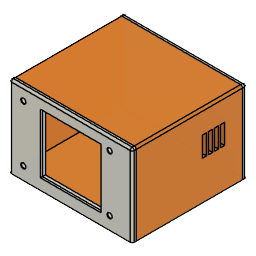
AirLog-E(together, no-placeholder-components) (Autodesk Fusion 360 design; units mm, degrees)
Autodesk Fusion 360 part; units mm, degrees
note: some values were not read from the file. Chosen so that the rebuilt part matches the saved one: which sketch regions a step uses; that a step has no effect.
sketch "Sketch1" plane through (0, 0, 0) normal (0, 1, 0) x (1, 0, 0)
  line L0 (24.9, -1.7) -> (-4.3, -1.7)
  line L1 (-4.3, -1.7) -> (-4.3, -30.3)
  line L2 (-4.3, -30.3) -> (24.9, -30.3)
  line L3 (24.9, -30.3) -> (24.9, -1.7)
  line L4 (30.9, 4.3) -> (-10.3, 4.3)
  line L5 (-10.3, -36.3) -> (30.9, -36.3)
  line L6 (-10.3, -36.3) -> (-20.3, -36.3)
  line L7 (-10.3, 4.3) -> (-20.3, 4.3)
  line L8 (30.9, -36.3) -> (40.9, -36.3)
  line L9 (30.9, 4.3) -> (40.9, 4.3)
  line L10 (40.9, -36.3) -> (40.9, 4.3)
  line L11 (-20.3, -36.3) -> (-20.3, 4.3)
  circle A0 centre (-13.355, -30.08) radius 1.08
  circle A1 centre (29.645, -30.08) radius 1.08
  circle A2 centre (-13.355, -2.08) radius 1.08
  circle A3 centre (29.645, -2.08) radius 1.08
  dimension "d2" = 6
  dimension "d3" = 10
  dimension "d4" = 10
  dimension "d5" = 10
  dimension "d6" = 10
  measures "d3" distance of L5.start L6.end
  measures "d4" distance of L4.end L7.end
  measures "d5" distance of L5.end L8.end
  measures "d6" distance of L4.start L9.end
extrude "Extrude1" add sketch "Sketch1" along normal blind 2 makes body 1
sketch "Sketch2" plane through (0, 0, 0) normal (0, 1, 0) x (1, 0, 0)
  circle A0 centre (29.635, -30.08) radius 1.0801
  circle A1 centre (-13.36, -30.08) radius 1.08
  circle A2 centre (-13.355, -2.08) radius 1.08
  circle A3 centre (29.6413, -2.0788) radius 1.0788
  line L0 (29.65, -29) -> (29.65, -28) construction
  line L1 (28.56, -30.08) -> (27.56, -30.08) construction
  line L2 (30.7151, -30.08) -> (31.7151, -30.08) construction
  line L3 (31.7151, -30.08) -> (31.7151, -28)
  line L4 (31.7151, -28) -> (29.65, -28)
  line L5 (27.56, -30.08) -> (27.56, -28)
  line L6 (27.56, -28) -> (29.65, -28)
  line L7 (27.56, -30.08) -> (27.56, -36.3)
  line L8 (31.7151, -30.08) -> (31.7151, -36.3)
  line L9 (31.7151, -36.3) -> (27.56, -36.3)
  line L10 (-15.44, -30.08) -> (-15.44, -36.3)
  line L11 (-15.44, -28) -> (-13.35, -28)
  line L12 (-11.2849, -36.3) -> (-15.44, -36.3)
  line L13 (-11.2849, -28) -> (-13.35, -28)
  line L14 (-14.44, -30.08) -> (-15.44, -30.08) construction
  line L15 (-11.2849, -30.08) -> (-11.2849, -36.3)
  line L16 (-13.35, -29) -> (-13.35, -28) construction
  circle A4 centre (-13.365, -30.08) radius 1.0801
  line L17 (-12.2849, -30.08) -> (-11.2849, -30.08) construction
  line L18 (-11.2849, -30.08) -> (-11.2849, -28)
  line L19 (-15.44, -30.08) -> (-15.44, -28)
  line L20 (-13.35, -3.15) -> (-13.35, -4.15) construction
  line L21 (-15.4151, -2.07) -> (-15.4151, 4.15)
  line L22 (-11.26, -2.07) -> (-11.26, 4.15)
  line L23 (-15.4151, -2.07) -> (-15.4151, -4.15)
  line L24 (-15.4151, -4.15) -> (-13.35, -4.15)
  line L25 (-11.26, -2.07) -> (-11.26, -4.15)
  line L26 (-14.4151, -2.07) -> (-15.4151, -2.07) construction
  line L27 (-11.26, -4.15) -> (-13.35, -4.15)
  circle A5 centre (-13.335, -2.07) radius 1.0801
  line L28 (-12.26, -2.07) -> (-11.26, -2.07) construction
  circle A6 centre (-13.34, -2.07) radius 1.08
  line L29 (28.5849, -2.07) -> (27.5849, -2.07) construction
  line L30 (31.74, -4.15) -> (29.65, -4.15)
  circle A7 centre (29.645, -2.08) radius 1.08
  line L31 (31.74, -2.07) -> (31.74, -4.15)
  line L32 (31.74, -2.07) -> (31.74, 4.15)
  line L33 (27.5849, -2.07) -> (27.5849, -4.15)
  line L34 (27.5849, -4.15) -> (29.65, -4.15)
  line L35 (30.74, -2.07) -> (31.74, -2.07) construction
  line L36 (27.5849, -2.07) -> (27.5849, 4.15)
  line L37 (29.65, -3.15) -> (29.65, -4.15) construction
  circle A8 centre (29.665, -2.07) radius 1.0801
  circle A9 centre (29.66, -2.07) radius 1.08
  line L38 (31.7151, -36.3) -> (40.9, -36.3)
  line L39 (40.9, -36.3) -> (40.9, 4.3)
  line L40 (40.9, 4.3) -> (-20.3, 4.3)
  line L41 (-20.3, 4.3) -> (-20.3, -36.3)
  line L42 (-20.3, -36.3) -> (27.56, -36.3)
  line L43 (31.74, 4.15) -> (31.74, 4.3)
  line L44 (27.5849, 4.15) -> (27.5849, 4.3)
  line L45 (-11.26, 4.15) -> (-11.26, 4.3)
  line L46 (-15.4151, 4.15) -> (-15.4151, 4.3)
  line L47 (31.7151, -33.8) -> (27.56, -33.8)
  line L48 (-17.8, -33.8) -> (27.56, -33.8)
  line L49 (-17.8, 1.8) -> (-17.8, -33.8)
  line L50 (38.4, 1.8) -> (-17.8, 1.8)
  line L51 (38.4, -33.8) -> (38.4, 1.8)
  line L52 (31.7151, -33.8) -> (38.4, -33.8)
  dimension "d9" = 1
  dimension "d10" = 1
  dimension "d11" = 1
  dimension "d12" = 1
  dimension "d13" = 1
  dimension "d14" = 1
  dimension "d15" = 1
  dimension "d16" = 1
  dimension "d17" = 2.5
  constraint coincident A0 L0.start
  constraint vertical L0
  constraint horizontal L1
  constraint coincident A0 L2.start
  constraint parallel L1 L2
  constraint perpendicular L2 L3
  constraint perpendicular L1 L5
  constraint perpendicular L0 L6
  constraint perpendicular L1 L7
  constraint perpendicular L2 L8
  constraint perpendicular L7 L9
  constraint coincident L16.start A4
  constraint vertical L16
  constraint horizontal L14
  constraint coincident L17.start A4
  constraint parallel L14 L17
  constraint perpendicular L17 L18
  constraint perpendicular L14 L19
  constraint perpendicular L11 L16
  constraint perpendicular L10 L14
  constraint perpendicular L15 L17
  constraint perpendicular L10 L12
  constraint coincident L20.start A5
  constraint coincident L26.start A5
  constraint parallel L26 L28
  constraint perpendicular L23 L26
  constraint perpendicular L25 L28
  constraint perpendicular L20 L27
  constraint perpendicular L22 L28
  constraint perpendicular L21 L26
  constraint coincident L37.start A8
  constraint coincident L29.start A8
  constraint parallel L29 L35
  constraint perpendicular L29 L33
  constraint perpendicular L31 L35
  constraint perpendicular L30 L37
  constraint perpendicular L32 L35
  constraint perpendicular L29 L36
  constraint perpendicular L8 L38
  constraint perpendicular L38 L39
  constraint perpendicular L21 L40
  constraint perpendicular L40 L41
  constraint perpendicular L7 L42
  constraint coincident L40 L43.end
  constraint perpendicular L40 L43
  constraint coincident L40 L44.end
  constraint perpendicular L40 L44
  constraint coincident L40 L45.end
  constraint perpendicular L40 L45
  constraint coincident L40 L46.end
  constraint perpendicular L40 L46
  measures "d9" distance of L1.start L1.end
  measures "d10" distance of L2.start L2.end
  measures "d11" distance of L10.start L14.start
  measures "d12" distance of L15.start L17.start
  measures "d13" distance of L22.start L28.start
  measures "d14" distance of L21.start L26.start
  measures "d15" distance of L31.start L35.start
  measures "d16" distance of L29.end L29.start
extrude "Extrude2" add sketch "Sketch2" along normal blind 50 separate body contours L3 L4 L5 L6 L7 L8 L47 | L8 L32 L38 L39 L40 L43 L50 L51 L52 | L7 L8 L9 L47 | L7 L15 L42 L48 | L10 L11 L13 L15 L18 L19 L48 | L10 L12 L15 L42 L48 | L10 L21 L40 L41 L42 L46 L48 L49 L50 | L32 L36 L40 L43 L44 L50 | L30 L31 L32 L33 L34 L36 L50 | L22 L36 L40 L44 L45 L50 | L21 L22 L40 L45 L46 L50 | L21 L22 L23 L24 L25 L27 L50 makes body 2
move_body "Move1" bodies 2 to x (1, 0, 0) y (0, 1, 0) z (0, 0, 1) at (0, 5, 0)
sketch "Sketch3" plane through (0, 5, 0) normal (0, -1, 0) x (1, 0, 0)
  line L0 (31.7151, 28) -> (31.7151, 33.8)
  line L1 (31.7151, 33.8) -> (38.4, 33.8)
  line L2 (38.4, 33.8) -> (38.4, -1.8)
  line L3 (38.4, -1.8) -> (31.74, -1.8)
  line L4 (31.74, -1.8) -> (31.74, 4.15)
  line L5 (31.74, 4.15) -> (29.65, 4.15)
  line L6 (29.65, 4.15) -> (27.5849, 4.15)
  line L7 (27.5849, 4.15) -> (27.5849, -1.8)
  line L8 (27.5849, -1.8) -> (-11.26, -1.8)
  line L9 (-11.26, -1.8) -> (-11.26, 4.15)
  line L10 (-11.26, 4.15) -> (-13.35, 4.15)
  line L11 (-13.35, 4.15) -> (-15.4151, 4.15)
  line L12 (-15.4151, 4.15) -> (-15.4151, -1.8)
  line L13 (-15.4151, -1.8) -> (-17.8, -1.8)
  line L14 (-17.8, -1.8) -> (-17.8, 33.8)
  line L15 (-17.8, 33.8) -> (-15.44, 33.8)
  line L16 (-15.44, 33.8) -> (-15.44, 28)
  line L17 (-15.44, 28) -> (-13.35, 28)
  line L18 (-13.35, 28) -> (-11.2849, 28)
  line L19 (-11.2849, 28) -> (-11.2849, 33.8)
  line L20 (-11.2849, 33.8) -> (27.56, 33.8)
  line L21 (27.56, 33.8) -> (27.56, 28)
  line L22 (27.56, 28) -> (29.65, 28)
  line L23 (29.65, 28) -> (31.7151, 28)
  circle A0 centre (29.635, 30.08) radius 1.0801
  arc A1 (-13.9461, 1.1761) -> (-13.36, 0.9902) centre (-13.34, 2.07) ccw
  arc A2 (-12.8659, 3.0429) -> (-13.9461, 1.1761) centre (-13.355, 2.08) ccw
  arc A3 (-13.36, 0.9902) -> (-12.8659, 3.0429) centre (-13.335, 2.07) ccw
  arc A4 (29.64, 0.9902) -> (30.1341, 3.0429) centre (29.665, 2.07) ccw
  arc A5 (29.1359, 1.1257) -> (29.64, 0.9902) centre (29.66, 2.07) ccw
  arc A6 (28.9927, 2.9408) -> (29.1359, 1.1257) centre (29.6413, 2.0788) ccw
  arc A7 (30.1341, 3.0429) -> (28.9927, 2.9408) centre (29.645, 2.08) ccw
  arc A8 (-13.34, 29.0002) -> (-13.34, 31.1598) centre (-13.36, 30.08) ccw
  arc A9 (-13.34, 31.1598) -> (-13.34, 29.0002) centre (-13.365, 30.08) ccw
  line L24 (40.9, 36.3) -> (-20.3, 36.3)
  line L25 (-20.3, 36.3) -> (-20.3, -4.3)
  line L26 (-20.3, -4.3) -> (40.9, -4.3)
  line L27 (40.9, -4.3) -> (40.9, 36.3)
  line L28 (-20.3, 36.3) -> (40.9, 36.3)
  line L29 (40.9, 36.3) -> (40.9, -4.3)
  line L30 (40.9, -4.3) -> (-20.3, -4.3)
  line L31 (-20.3, -4.3) -> (-20.3, 36.3)
  line L32 (38.4, -1.8) -> (-17.8, -1.8)
  line L33 (-17.8, -1.8) -> (-17.8, 33.8)
  line L34 (-17.8, 33.8) -> (38.4, 33.8)
  line L35 (38.4, 33.8) -> (38.4, -1.8)
  constraint horizontal L28
  constraint vertical L29
  constraint horizontal L30
  constraint vertical L31
  constraint coincident L26.end L27.start
  constraint coincident L24.end L25.start
  constraint horizontal L32
  constraint vertical L33
  constraint horizontal L34
  constraint vertical L35
  constraint coincident L14.end L15.start
  constraint coincident L2.end L3.start
extrude "Extrude3" add sketch "Sketch3" along normal blind 3 contours L24 L25 L26 L27 L28 L29 L30 L31 bodies 2
sketch "Sketch4" plane through (0, 55, 0) normal (0, 1, 0) x (-1, 0, 0)
  line L0 (-31.7151, 33.8) -> (-31.7151, 28)
  line L1 (-31.7151, 28) -> (-29.65, 28)
  line L2 (-29.65, 28) -> (-27.56, 28)
  line L3 (-27.56, 28) -> (-27.56, 33.8)
  line L4 (-27.56, 33.8) -> (11.2849, 33.8)
  line L5 (11.2849, 33.8) -> (11.2849, 28)
  line L6 (11.2849, 28) -> (13.35, 28)
  line L7 (13.35, 28) -> (15.44, 28)
  line L8 (15.44, 28) -> (15.44, 33.8)
  line L9 (15.44, 33.8) -> (17.8, 33.8)
  line L10 (17.8, 33.8) -> (17.8, -1.8)
  line L11 (17.8, -1.8) -> (15.4151, -1.8)
  line L12 (15.4151, -1.8) -> (15.4151, 4.15)
  line L13 (15.4151, 4.15) -> (13.35, 4.15)
  line L14 (13.35, 4.15) -> (11.26, 4.15)
  line L15 (11.26, 4.15) -> (11.26, -1.8)
  line L16 (11.26, -1.8) -> (-27.5849, -1.8)
  line L17 (-27.5849, -1.8) -> (-27.5849, 4.15)
  line L18 (-27.5849, 4.15) -> (-29.65, 4.15)
  line L19 (-29.65, 4.15) -> (-31.74, 4.15)
  line L20 (-31.74, 4.15) -> (-31.74, -1.8)
  line L21 (-31.74, -1.8) -> (-38.4, -1.8)
  line L22 (-38.4, -1.8) -> (-38.4, 33.8)
  line L23 (-38.4, 33.8) -> (-31.7151, 33.8)
  circle A0 centre (-29.635, 30.08) radius 1.0801
  arc A1 (13.36, 0.9902) -> (13.9461, 1.1761) centre (13.34, 2.07) ccw
  arc A2 (12.8659, 3.0429) -> (13.36, 0.9902) centre (13.335, 2.07) ccw
  arc A3 (13.9461, 1.1761) -> (12.8659, 3.0429) centre (13.355, 2.08) ccw
  arc A4 (-30.1341, 3.0429) -> (-29.64, 0.9902) centre (-29.665, 2.07) ccw
  arc A5 (-28.9927, 2.9408) -> (-30.1341, 3.0429) centre (-29.645, 2.08) ccw
  arc A6 (-29.1359, 1.1257) -> (-28.9927, 2.9408) centre (-29.6413, 2.0788) ccw
  arc A7 (-29.64, 0.9902) -> (-29.1359, 1.1257) centre (-29.66, 2.07) ccw
  arc A8 (13.34, 31.1598) -> (13.34, 29.0002) centre (13.36, 30.08) ccw
  arc A9 (13.34, 29.0002) -> (13.34, 31.1598) centre (13.365, 30.08) ccw
  line L24 (20.3, 36.3) -> (-40.9, 36.3)
  line L25 (-40.9, 36.3) -> (-40.9, -4.3)
  line L26 (-40.9, -4.3) -> (20.3, -4.3)
  line L27 (20.3, -4.3) -> (20.3, 36.3)
  line L28 (-31.7151, 33.8) -> (-27.56, 33.8)
  line L29 (-27.56, 33.8) -> (-27.56, 28)
  line L30 (-27.56, 28) -> (-31.7151, 28)
  line L31 (-31.7151, 28) -> (-31.7151, 33.8)
  line L32 (11.2849, 33.8) -> (15.44, 33.8)
  line L33 (15.44, 33.8) -> (15.44, 28)
  line L34 (15.44, 28) -> (11.2849, 28)
  line L35 (11.2849, 28) -> (11.2849, 33.8)
  line L36 (11.26, 4.15) -> (15.4151, 4.15)
  line L37 (15.4151, 4.15) -> (15.4151, -1.8)
  line L38 (15.4151, -1.8) -> (11.26, -1.8)
  line L39 (11.26, -1.8) -> (11.26, 4.15)
  line L40 (-31.74, 4.15) -> (-27.5849, 4.15)
  line L41 (-27.5849, 4.15) -> (-27.5849, -1.8)
  line L42 (-27.5849, -1.8) -> (-31.74, -1.8)
  line L43 (-31.74, -1.8) -> (-31.74, 4.15)
  constraint horizontal L28
  constraint vertical L29
  constraint horizontal L30
  constraint vertical L31
  constraint coincident L2.end L3.start
  constraint coincident L0.start L23.end
  constraint horizontal L32
  constraint vertical L33
  constraint horizontal L34
  constraint vertical L35
  constraint coincident L7.end L8.start
  constraint coincident L4.end L5.start
  constraint horizontal L36
  constraint vertical L37
  constraint horizontal L38
  constraint vertical L39
  constraint coincident L11.end L12.start
  constraint coincident L14.end L15.start
  constraint horizontal L40
  constraint vertical L41
  constraint horizontal L42
  constraint vertical L43
  constraint coincident L16.end L17.start
  constraint coincident L19.end L20.start
extrude "Extrude4" cut sketch "Sketch4" against normal blind 48 contours L0 L1 L2 L3 L28 L29 L30 L31 | L5 L6 L7 L8 L32 L33 L34 L35 | L17 L18 L19 L20 L40 L41 L42 L43 | L12 L13 L14 L15 L36 L37 L38 L39 | A0 | A1 A2 A3 | A4 A5 A6 A7 | A8 A9 bodies 2
chamfer "Chamfer1" distance 0.2 angle 45 10 edges at (-12.28, 5, 30.08) (-14.4451, 5, 30.08) (28.628, 5, 29.6894) (30.7151, 5, 1.8172) (28.5658, 5, 1.9939) (29.3796, 5, 1.027) (29.5487, 5, 3.1557) (-12.2849, 5, 1.8172) (-13.6665, 5, 1.0405) (-14.2898, 5, 2.6209) on bodies 2
chamfer "Chamfer2" distance 0.2 angle 45 4 edges at (-14.3619, 0, 29.6895) (28.6381, 0, 1.6895) (28.6381, 0, 29.6895) (-14.3619, 0, 1.6895) on bodies 1
chamfer "Chamfer3" distance 0.5 angle 45 4 edges at (-4.3, 0, 16) (10.3, 0, 30.3) (10.3, 0, 1.7) (24.9, 0, 16) on bodies 1
sketch "Sketch5" plane through (0, 0, 0) normal (0, 0, 1) x (1, 0, 0)
  line L0 (20, -25) -> (-30, -25)
  line L1 (-30, -25) -> (-30, 9)
  line L2 (-30, 9) -> (20, 9)
  line L3 (20, 9) -> (20, -25)
  dimension "d27" = 34
  constraint horizontal L0
  constraint vertical L1
  constraint horizontal L2
  constraint vertical L3
  measures "d27" distance of L0.start L2.end
sketch "Sketch6" plane through (0, 0, 10) normal (0, 0, 1) x (-1, 0, 0)
  line L0 (-17, 21) -> (-17, -5)
  line L1 (-17, -5) -> (27, -5)
  line L2 (27, -5) -> (27, 21)
  line L3 (27, 21) -> (-17, 21)
  line L4 (12.4645, 11) -> (-7, 11) construction
  line L5 (-7, 11) -> (-7, 4.44) construction
  line L6 (-7, 4.44) -> (12.4645, 4.44) construction
  line L7 (12.4645, 4.44) -> (12.4645, 11) construction
  dimension "d38" = 2
sketch "Sketch7" plane through (-17.8, 0, 0) normal (1, 0, 0) x (0, 1, 0)
  line L0 (2, -1.8) -> (55, -1.8)
  line L1 (55, -1.8) -> (55, 33.8)
  line L2 (55, 33.8) -> (2, 33.8)
  line L3 (2, 33.8) -> (2, -1.8)
  line L4 (30, 25) -> (32, 25)
  line L5 (32, 25) -> (32, 20)
  line L6 (32, 20) -> (30, 20)
  line L7 (30, 20) -> (30, 25)
  constraint horizontal L4
  constraint vertical L5
  constraint horizontal L6
  constraint vertical L7
extrude "Extrude7" add sketch "Sketch7" along normal blind 8 contours L4 L5 L6 L7 bodies 2
sketch "Sketch8" plane through (0, 32, 0) normal (0, 1, 0) x (-1, 0, 0)
  line L0 (17.8, 20) -> (17.8, 25)
  line L1 (17.8, 25) -> (9.8, 25)
  line L2 (9.8, 25) -> (9.8, 20)
  line L3 (9.8, 20) -> (17.8, 20)
  circle A0 centre (13.5, 22.5) radius 1.25
  dimension "d44" = 2.5
  measures "d44" diameter of A0
extrude "Extrude8" cut sketch "Sketch8" against normal blind 2 contours A0 bodies 2
sketch "Sketch9" plane through (38.4, 0, 0) normal (-1, 0, 0) x (0, -1, 0)
  line L0 (-2, 33.8) -> (-55, 33.8)
  line L1 (-55, 33.8) -> (-55, -1.8)
  line L2 (-55, -1.8) -> (-2, -1.8)
  line L3 (-2, -1.8) -> (-2, 33.8)
  line L4 (-30, 25) -> (-30, 20)
  line L5 (-30, 20) -> (-32, 20)
  line L6 (-32, 25) -> (-30, 25)
  line L7 (-32, 20) -> (-32, 25)
  constraint horizontal L6
  constraint vertical L4
  constraint horizontal L5
  constraint vertical L7
extrude "Extrude9" add sketch "Sketch9" along normal blind 8 contours L4 L5 L6 L7 bodies 2
sketch "Sketch10" plane through (0, 32, 0) normal (0, 1, 0) x (-1, 0, 0)
  line L0 (-38.4, 25) -> (-38.4, 20)
  line L1 (-38.4, 20) -> (-30.4, 20)
  line L2 (-30.4, 20) -> (-30.4, 25)
  line L3 (-30.4, 25) -> (-38.4, 25)
  circle A0 centre (-34.1, 22.5) radius 1.25
  dimension "d51" = 2.5
  measures "d51" diameter of A0
extrude "Extrude10" cut sketch "Sketch10" against normal blind 2 contours A0 bodies 2
sketch "Sketch11" plane through (-20.3, 0, 0) normal (-1, 0, 0) x (0, -1, 0)
  line L0 (-2, 36.3) -> (-55, 36.3)
  line L1 (-55, 36.3) -> (-55, -4.3)
  line L2 (-55, -4.3) -> (-2, -4.3)
  line L3 (-2, -4.3) -> (-2, 36.3)
  line L4 (-35, 25) -> (-37, 25)
  line L5 (-37, 25) -> (-37, 15)
  line L6 (-37, 15) -> (-35, 15)
  line L7 (-35, 15) -> (-35, 25)
  line L8 (-38, 25) -> (-40, 25)
  line L9 (-40, 25) -> (-40, 15)
  line L10 (-40, 15) -> (-38, 15)
  line L11 (-38, 15) -> (-38, 25)
  line L12 (-41, 25) -> (-43, 25)
  line L13 (-43, 25) -> (-43, 15)
  line L14 (-43, 15) -> (-41, 15)
  line L15 (-41, 15) -> (-41, 25)
  line L16 (-44, 25) -> (-46, 25)
  line L17 (-46, 25) -> (-46, 15)
  line L18 (-46, 15) -> (-44, 15)
  line L19 (-44, 15) -> (-44, 25)
  dimension "d54" = 2
  dimension "d55" = 10
  dimension "d56" = 2
  dimension "d57" = 10
  dimension "d58" = 2
  dimension "d59" = 10
  dimension "d60" = 2
  dimension "d61" = 10
  constraint horizontal L4
  constraint vertical L5
  constraint horizontal L6
  constraint vertical L7
  constraint horizontal L8
  constraint vertical L9
  constraint horizontal L10
  constraint vertical L11
  constraint horizontal L12
  constraint vertical L13
  constraint horizontal L14
  constraint vertical L15
  constraint horizontal L16
  constraint vertical L17
  constraint horizontal L18
  constraint vertical L19
  measures "d54" distance of L4.start L4.end
  measures "d55" distance of L4.start L6.end
  measures "d56" distance of L8.start L8.end
  measures "d57" distance of L8.start L10.end
  measures "d58" distance of L12.start L12.end
  measures "d59" distance of L12.start L14.end
  measures "d60" distance of L16.start L16.end
  measures "d61" distance of L16.start L18.end
sketch "Sketch12" plane through (40.9, 0, 0) normal (1, 0, 0) x (0, 1, 0)
  line L0 (2, -4.3) -> (55, -4.3)
  line L1 (55, -4.3) -> (55, 36.3)
  line L2 (55, 36.3) -> (2, 36.3)
  line L3 (2, 36.3) -> (2, -4.3)
  line L4 (41, 25) -> (41, 15)
  line L5 (46, 25) -> (44, 25)
  line L6 (40, 15) -> (40, 25)
  line L7 (43, 15) -> (43, 25)
  line L8 (41, 15) -> (43, 15)
  line L9 (43, 25) -> (41, 25)
  line L10 (37, 25) -> (35, 25)
  line L11 (38, 25) -> (38, 15)
  line L12 (37, 15) -> (37, 25)
  line L13 (46, 15) -> (46, 25)
  line L14 (38, 15) -> (40, 15)
  line L15 (35, 25) -> (35, 15)
  line L16 (44, 15) -> (46, 15)
  line L17 (44, 25) -> (44, 15)
  line L18 (35, 15) -> (37, 15)
  line L19 (40, 25) -> (38, 25)
  dimension "d62" = 2
  dimension "d63" = 10
  dimension "d64" = 2
  dimension "d65" = 10
  dimension "d66" = 2
  dimension "d67" = 10
  dimension "d68" = 2
  dimension "d69" = 10
  constraint horizontal L5
  constraint vertical L17
  constraint horizontal L16
  constraint vertical L13
  constraint horizontal L9
  constraint vertical L4
  constraint horizontal L8
  constraint vertical L7
  constraint horizontal L19
  constraint vertical L11
  constraint horizontal L14
  constraint vertical L6
  constraint horizontal L10
  constraint vertical L15
  constraint horizontal L18
  constraint vertical L12
  measures "d62" distance of L5.end L5.start
  measures "d63" distance of L5.start L13.start
  measures "d64" distance of L7.end L4.start
  measures "d65" distance of L7.end L7.start
  measures "d66" distance of L11.start L6.end
  measures "d67" distance of L6.start L6.end
  measures "d68" distance of L10.start L10.end
  measures "d69" distance of L10.start L12.start
extrude "Extrude11" cut sketch "Sketch11" against normal blind 2.5 contours L4 L5 L6 L7 | L8 L9 L10 L11 | L12 L13 L14 L15 | L16 L17 L18 L19 bodies 2
extrude "Extrude12" cut sketch "Sketch12" against normal blind 2.5 contours L4 L7 L8 L9 | L5 L13 L16 L17 | L6 L11 L14 L19 | L10 L12 L15 L18 bodies 2
sketch "Sketch13" plane through (0, 0, 0) normal (0, 1, 0) x (1, 0, 0)
  line L0 (40.9, -36.3, 55) -> (-20.3, -36.3, 55)
  line L1 (-20.3, -36.3, 55) -> (-20.3, 4.3, 55)
  line L2 (-20.3, 4.3, 55) -> (40.9, 4.3, 55)
  line L3 (40.9, 4.3, 55) -> (40.9, -36.3, 55)
  line L4 (31.7151, -36.3, 55) -> (27.56, -36.3, 55)
  line L5 (29.65, -29, 55) -> (29.65, -28, 55) construction
  line L6 (27.5849, 4.15, 55) -> (27.5849, 4.3, 55)
  line L7 (30.74, -2.07, 55) -> (31.74, -2.07, 55) construction
  line L8 (29.65, -3.15, 55) -> (29.65, -4.15, 55) construction
  line L9 (-17.8, -33.8, 55) -> (27.56, -33.8, 55)
  line L10 (-14.4151, -2.07, 55) -> (-15.4151, -2.07, 55) construction
  line L11 (-13.35, -29, 55) -> (-13.35, -28, 55) construction
  line L12 (-14.44, -30.08, 55) -> (-15.44, -30.08, 55) construction
  line L13 (28.56, -30.08, 55) -> (27.56, -30.08, 55) construction
  line L14 (-11.2849, -36.3, 55) -> (-15.44, -36.3, 55)
  line L15 (30.7151, -30.08, 55) -> (31.7151, -30.08, 55) construction
  line L16 (40.9, 4.3, 55) -> (-20.3, 4.3, 55)
  line L17 (38.4, 1.8, 55) -> (-17.8, 1.8, 55)
  line L18 (-20.3, 4.3, 55) -> (-20.3, -36.3, 55)
  line L19 (-12.26, -2.07, 55) -> (-11.26, -2.07, 55) construction
  line L20 (-15.4151, 4.15, 55) -> (-15.4151, 4.3, 55)
  line L21 (-11.26, 4.15, 55) -> (-11.26, 4.3, 55)
  line L22 (-12.2849, -30.08, 55) -> (-11.2849, -30.08, 55) construction
  line L23 (-13.35, -3.15, 55) -> (-13.35, -4.15, 55) construction
  line L24 (-20.3, -36.3, 55) -> (27.56, -36.3, 55)
  line L25 (-17.8, 1.8, 55) -> (-17.8, -33.8, 55)
  line L26 (38.4, -33.8, 55) -> (38.4, 1.8, 55)
  line L27 (31.7151, -33.8, 55) -> (38.4, -33.8, 55)
  line L28 (31.7151, -33.8, 55) -> (27.56, -33.8, 55)
  line L29 (31.74, 4.15, 55) -> (31.74, 4.3, 55)
  line L30 (28.5849, -2.07, 55) -> (27.5849, -2.07, 55) construction
  line L31 (40.9, -36.3, 55) -> (40.9, 4.3, 55)
  line L32 (31.7151, -36.3, 55) -> (40.9, -36.3, 55)
  circle A0 through (31.635, -30.08, 55) (28.635, -28.348, 55) (28.635, -31.8121, 55)
  circle A1 through (-11.365, -30.08, 55) (-14.365, -28.348, 55) (-14.365, -31.8121, 55)
  circle A2 through (-11.34, -2.07, 55) (-14.34, -0.3379, 55) (-14.34, -3.802, 55)
  circle A3 through (31.645, -2.08, 55) (28.645, -0.3479, 55) (28.645, -3.8121, 55)
  line L33 (31.74, -1.2617, 55) -> (33.24, -1.2617, 55) construction
  line L34 (27.5849, -1.1744, 55) -> (26.0849, -1.1744, 55) construction
  line L35 (29.65, -4.15, 55) -> (29.65, -5.65, 55) construction
  line L36 (33.24, -1.2617, 55) -> (33.24, 1.8, 55)
  line L37 (26.0849, -1.1744, 55) -> (26.0849, 1.8, 55)
  line L38 (29.65, -5.65, 55) -> (33.24, -5.65, 55)
  line L39 (29.65, -5.65, 55) -> (26.0849, -5.65, 55)
  line L40 (26.0849, -5.65, 55) -> (26.0849, -1.1744, 55)
  line L41 (33.24, -5.65, 55) -> (33.24, -1.2617, 55)
  line L42 (-13.35, -4.07, 55) -> (-13.35, -5.57, 55) construction
  line L43 (-15.34, -2.07, 55) -> (-16.84, -2.07, 55) construction
  line L44 (-11.26, -2.07, 55) -> (-9.76, -2.07, 55) construction
  line L45 (-13.35, -5.57, 55) -> (-9.76, -5.57, 55)
  line L46 (-13.35, -5.57, 55) -> (-16.84, -5.57, 55)
  line L47 (-16.84, -5.57, 55) -> (-16.84, 1.8, 55)
  line L48 (-9.76, -5.57, 55) -> (-9.76, 1.8, 55)
  line L49 (-11.365, -30.08, 55) -> (-9.865, -30.08, 55) construction
  line L50 (-15.365, -30.08, 55) -> (-16.865, -30.08, 55) construction
  line L51 (-13.35, -28.0801, 55) -> (-13.35, -26.5801, 55) construction
  line L52 (-16.865, -30.08, 55) -> (-16.865, -30, 55) construction
  line L53 (-9.865, -30.08, 55) -> (-9.865, -33.8, 55)
  line L54 (-16.865, -30.08, 55) -> (-16.865, -33.8, 55)
  line L55 (-13.35, -26.5801, 55) -> (-16.865, -26.5801, 55)
  line L56 (-13.35, -26.5801, 55) -> (-9.865, -26.5801, 55)
  line L57 (-9.865, -26.5801, 55) -> (-9.865, -29.5, 55)
  line L58 (-16.865, -26.5801, 55) -> (-16.865, -30.08, 55)
  line L59 (27.635, -30.08, 55) -> (26.135, -30.08, 55) construction
  line L60 (31.635, -30.08, 55) -> (33.135, -30.08, 55) construction
  line L61 (29.65, -28.0801, 55) -> (29.65, -26.5801, 55) construction
  line L62 (26.135, -30.08, 55) -> (26.135, -33.8, 55)
  line L63 (33.135, -30.08, 55) -> (33.135, -33.8, 55)
  line L64 (29.65, -26.5801, 55) -> (33.135, -26.5801, 55)
  line L65 (29.65, -26.5801, 55) -> (26.135, -26.5801, 55)
  line L66 (26.135, -26.5801, 55) -> (26.135, -30.08, 55)
  line L67 (33.135, -26.5801, 55) -> (33.135, -30.08, 55)
  line L68 (-9.865, -29.5, 55) -> (-9.865, -30.08, 55)
  dimension "d75" = 1
  dimension "d76" = 1
  dimension "d77" = 1
  dimension "d78" = 1
  dimension "d79" = 1
  dimension "d80" = 1
  dimension "d81" = 1
  dimension "d82" = 1
  dimension "d85" = 4
  dimension "d86" = 4
  dimension "d87" = 4
  dimension "d88" = 4
  dimension "d89" = 1.5
  dimension "d90" = 1.5
  dimension "d91" = 1.5
  dimension "d92" = 1.5
  dimension "d93" = 1.5
  dimension "d94" = 1.5
  dimension "d95" = 1.5
  dimension "d96" = 1.5
  dimension "d97" = 1.5
  dimension "d98" = 1.5
  dimension "d99" = 1.5
  dimension "d100" = 1.5
combine "Combine1" [no effect]
sketch "Sketch13 (curves 55 mm off its plane)" plane through (0, 55, 0) normal (0, 1, 0) x (1, 0, 0)
  line L0 (40.9, -36.3) -> (-20.3, -36.3)
  line L1 (-20.3, -36.3) -> (-20.3, 4.3)
  line L2 (-20.3, 4.3) -> (40.9, 4.3)
  line L3 (40.9, 4.3) -> (40.9, -36.3)
  line L4 (31.7151, -36.3) -> (27.56, -36.3)
  line L5 (29.65, -29) -> (29.65, -28) construction
  line L6 (27.5849, 4.15) -> (27.5849, 4.3)
  line L7 (30.74, -2.07) -> (31.74, -2.07) construction
  line L8 (29.65, -3.15) -> (29.65, -4.15) construction
  line L9 (-17.8, -33.8) -> (27.56, -33.8)
  line L10 (-14.4151, -2.07) -> (-15.4151, -2.07) construction
  line L11 (-13.35, -29) -> (-13.35, -28) construction
  line L12 (-14.44, -30.08) -> (-15.44, -30.08) construction
  line L13 (28.56, -30.08) -> (27.56, -30.08) construction
  line L14 (-11.2849, -36.3) -> (-15.44, -36.3)
  line L15 (30.7151, -30.08) -> (31.7151, -30.08) construction
  line L16 (40.9, 4.3) -> (-20.3, 4.3)
  line L17 (38.4, 1.8) -> (-17.8, 1.8)
  line L18 (-20.3, 4.3) -> (-20.3, -36.3)
  line L19 (-12.26, -2.07) -> (-11.26, -2.07) construction
  line L20 (-15.4151, 4.15) -> (-15.4151, 4.3)
  line L21 (-11.26, 4.15) -> (-11.26, 4.3)
  line L22 (-12.2849, -30.08) -> (-11.2849, -30.08) construction
  line L23 (-13.35, -3.15) -> (-13.35, -4.15) construction
  line L24 (-20.3, -36.3) -> (27.56, -36.3)
  line L25 (-17.8, 1.8) -> (-17.8, -33.8)
  line L26 (38.4, -33.8) -> (38.4, 1.8)
  line L27 (31.7151, -33.8) -> (38.4, -33.8)
  line L28 (31.7151, -33.8) -> (27.56, -33.8)
  line L29 (31.74, 4.15) -> (31.74, 4.3)
  line L30 (28.5849, -2.07) -> (27.5849, -2.07) construction
  line L31 (40.9, -36.3) -> (40.9, 4.3)
  line L32 (31.7151, -36.3) -> (40.9, -36.3)
  circle A0 centre (29.635, -30.08) radius 2
  circle A1 centre (-13.365, -30.08) radius 2
  circle A2 centre (-13.34, -2.07) radius 2
  circle A3 centre (29.645, -2.08) radius 2
  line L33 (31.74, -1.2617) -> (33.24, -1.2617) construction
  line L34 (27.5849, -1.1744) -> (26.0849, -1.1744) construction
  line L35 (29.65, -4.15) -> (29.65, -5.65) construction
  line L36 (33.24, -1.2617) -> (33.24, 1.8)
  line L37 (26.0849, -1.1744) -> (26.0849, 1.8)
  line L38 (29.65, -5.65) -> (33.24, -5.65)
  line L39 (29.65, -5.65) -> (26.0849, -5.65)
  line L40 (26.0849, -5.65) -> (26.0849, -1.1744)
  line L41 (33.24, -5.65) -> (33.24, -1.2617)
  line L42 (-13.35, -4.07) -> (-13.35, -5.57) construction
  line L43 (-15.34, -2.07) -> (-16.84, -2.07) construction
  line L44 (-11.26, -2.07) -> (-9.76, -2.07) construction
  line L45 (-13.35, -5.57) -> (-9.76, -5.57)
  line L46 (-13.35, -5.57) -> (-16.84, -5.57)
  line L47 (-16.84, -5.57) -> (-16.84, 1.8)
  line L48 (-9.76, -5.57) -> (-9.76, 1.8)
  line L49 (-11.365, -30.08) -> (-9.865, -30.08) construction
  line L50 (-15.365, -30.08) -> (-16.865, -30.08) construction
  line L51 (-13.35, -28.0801) -> (-13.35, -26.5801) construction
  line L52 (-16.865, -30.08) -> (-16.865, -30) construction
  line L53 (-9.865, -30.08) -> (-9.865, -33.8)
  line L54 (-16.865, -30.08) -> (-16.865, -33.8)
  line L55 (-13.35, -26.5801) -> (-16.865, -26.5801)
  line L56 (-13.35, -26.5801) -> (-9.865, -26.5801)
  line L57 (-9.865, -26.5801) -> (-9.865, -29.5)
  line L58 (-16.865, -26.5801) -> (-16.865, -30.08)
  line L59 (27.635, -30.08) -> (26.135, -30.08) construction
  line L60 (31.635, -30.08) -> (33.135, -30.08) construction
  line L61 (29.65, -28.0801) -> (29.65, -26.5801) construction
  line L62 (26.135, -30.08) -> (26.135, -33.8)
  line L63 (33.135, -30.08) -> (33.135, -33.8)
  line L64 (29.65, -26.5801) -> (33.135, -26.5801)
  line L65 (29.65, -26.5801) -> (26.135, -26.5801)
  line L66 (26.135, -26.5801) -> (26.135, -30.08)
  line L67 (33.135, -26.5801) -> (33.135, -30.08)
  line L68 (-9.865, -29.5) -> (-9.865, -30.08)
extrude "Extrude14" add sketch "Sketch13 (curves 55 mm off its plane)" against normal blind 7 contours L9 L53 L54 L55 L56 L57 L58 L68 | L17 L45 L46 L47 L48 | L9 L27 L28 L62 L63 L64 L65 L66 L67 | L17 L36 L37 L38 L39 L40 L41 bodies 2
sketch "Sketch14" plane through (0, 48, 0) normal (0, -1, 0) x (1, 0, 0)
  circle A0 centre (29.635, 30.08) radius 2
  line L0 (26.135, 26.5801) -> (33.135, 26.5801)
  line L1 (33.135, 26.5801) -> (33.135, 33.8)
  line L2 (33.135, 33.8) -> (26.135, 33.8)
  line L3 (26.135, 33.8) -> (26.135, 26.5801)
  line L4 (-9.865, 26.58) -> (-16.865, 26.58)
  line L5 (-16.865, 26.58) -> (-16.865, 33.8)
  line L6 (-16.865, 33.8) -> (-9.865, 33.8)
  line L7 (-9.865, 33.8) -> (-9.865, 26.58)
  line L8 (26.135, 33.8) -> (33.135, 33.8)
  line L9 (33.135, 33.8) -> (33.135, 26.5801)
  line L10 (33.135, 26.5801) -> (26.135, 26.5801)
  line L11 (26.135, 26.5801) -> (26.135, 33.8)
  line L12 (26.085, 5.65) -> (33.24, 5.65)
  line L13 (33.24, 5.65) -> (33.24, -1.8)
  line L14 (33.24, -1.8) -> (26.085, -1.8)
  line L15 (26.085, -1.8) -> (26.085, 5.65)
  line L16 (-16.84, -1.8) -> (-9.76, -1.8)
  line L17 (-9.76, -1.8) -> (-9.76, 5.57)
  line L18 (-9.76, 5.57) -> (-16.84, 5.57)
  line L19 (-16.84, 5.57) -> (-16.84, -1.8)
  constraint horizontal L4
  constraint vertical L5
  constraint horizontal L6
  constraint vertical L7
  constraint horizontal L8
  constraint vertical L9
  constraint horizontal L10
  constraint vertical L11
  constraint coincident L0.end L1.start
  constraint coincident L2.end L3.start
  constraint horizontal L12
  constraint vertical L13
  constraint horizontal L14
  constraint vertical L15
  constraint horizontal L16
  constraint vertical L17
  constraint horizontal L18
  constraint vertical L19
extrude "Extrude15" add sketch "Sketch14" along normal blind 2 contours A0 | L0 L1 L2 L3 L8 L9 L10 L11 | L4 L5 L6 L7 | L12 L13 L14 L15 | L16 L17 L18 L19 bodies 2
chamfer "Chamfer4" distance 0.2 angle 45 4 edges at (27.7703, 55, 29.3568) (-15.2297, 55, 29.3568) (-15.2047, 55, 1.3468) (27.7803, 55, 1.3568) on bodies 2
sketch "Sketch15" plane through (0, 55, 0) normal (0, 1, 0) x (-1, 0, 0)
  circle A0 centre (13.34, 2.07) radius 2.2
  circle A1 centre (-29.635, 30.08) radius 2.2
  line L0 (-38.4, 33.8) -> (-33.135, 33.8)
  line L1 (-33.135, 33.8) -> (-33.135, 26.5801)
  line L2 (-33.135, 26.5801) -> (-26.135, 26.5801)
  line L3 (-26.135, 26.5801) -> (-26.135, 33.8)
  line L4 (-26.135, 33.8) -> (9.865, 33.8)
  line L5 (9.865, 33.8) -> (9.865, 26.5801)
  line L6 (9.865, 26.5801) -> (16.865, 26.5801)
  line L7 (16.865, 26.5801) -> (16.865, 33.8)
  line L8 (16.865, 33.8) -> (17.8, 33.8)
  line L9 (17.8, 33.8) -> (17.8, -1.8)
  line L10 (17.8, -1.8) -> (16.84, -1.8)
  line L11 (16.84, -1.8) -> (16.84, 5.57)
  line L12 (16.84, 5.57) -> (9.76, 5.57)
  line L13 (9.76, 5.57) -> (9.76, -1.8)
  line L14 (9.76, -1.8) -> (-26.0849, -1.8)
  line L15 (-26.0849, -1.8) -> (-26.0849, 5.65)
  line L16 (-26.0849, 5.65) -> (-33.24, 5.65)
  line L17 (-33.24, 5.65) -> (-33.24, -1.8)
  line L18 (-33.24, -1.8) -> (-38.4, -1.8)
  line L19 (-38.4, -1.8) -> (-38.4, 33.8)
  line L20 (20.3, 36.3) -> (-40.9, 36.3)
  line L21 (-40.9, 36.3) -> (-40.9, -4.3)
  line L22 (-40.9, -4.3) -> (20.3, -4.3)
  line L23 (20.3, -4.3) -> (20.3, 36.3)
  circle A2 centre (13.365, 30.08) radius 2.2
  circle A3 centre (-29.645, 2.08) radius 2.2
  line L24 (-40.9, 36.3) -> (20.3, 36.3)
  line L25 (20.3, 36.3) -> (20.3, -4.3)
  line L26 (20.3, -4.3) -> (-40.9, -4.3)
  line L27 (-40.9, -4.3) -> (-40.9, 36.3)
  line L28 (-29.64, 32.08) -> (-29.64, 28.08) construction
  circle A4 centre (-29.635, 30.08) radius 1.6
  circle A5 centre (13.365, 30.08) radius 1.6
  circle A6 centre (13.34, 2.07) radius 1.6
  circle A7 centre (-29.645, 2.08) radius 1.6
  dimension "d106" = 3.2
  dimension "d107" = 3.2
  dimension "d108" = 3.2
  dimension "d109" = 3.2
  constraint horizontal L24
  constraint vertical L25
  constraint horizontal L26
  constraint vertical L27
  constraint coincident L22.end L23.start
  constraint coincident L20.end L21.start
  constraint vertical L28
  constraint concentric A1 A4
  constraint concentric A2 A5
  constraint concentric A0 A6
  constraint concentric A3 A7
  measures "d106" diameter of A4
  measures "d107" diameter of A5
  measures "d108" diameter of A6
  measures "d109" diameter of A7
extrude "Extrude16" add sketch "Sketch15" along normal blind 2 separate body contours L0 L1 L2 L3 L4 L5 L6 L7 L8 L9 L10 L11 L12 L13 L14 L15 L16 L17 L18 L19 | L20 L21 L22 L23 L24 L25 L26 L27 makes body 3
chamfer "Chamfer5" distance 0.5 angle 45 4 edges at (31.6861, 57, 30.8756) (31.6961, 57, 2.8756) (-11.2889, 57, 2.8656) (-11.3139, 57, 30.8756) on bodies 3
sketch "Sketch16" plane through (0, 0, 36.3) normal (0, 0, 1) x (-1, 0, 0)
  line L0 (-40.9, -2) -> (-40.9, -55)
  line L1 (-40.9, -55) -> (20.3, -55)
  line L2 (20.3, -55) -> (20.3, -2)
  line L3 (20.3, -2) -> (-40.9, -2)
  line L4 (-87.4118, -33.3412, -35) -> (-51.548, -33.3602, -35) construction
  line L5 (-51.548, -33.3602, -35) -> (-51.5354, -9.6159, -35) construction
  line L6 (-51.5354, -9.6159, -35) -> (-87.3992, -9.5969, -35) construction
  line L7 (-87.3992, -9.5969, -35) -> (-87.4118, -33.3412, -35) construction
  dimension "d113" = 2
fillet "Fillet5" radius 1 5 edges at (-20.3, 1, 36.3) (10.3, 0, 36.3) (40.9, 1, 36.3) (40.9, 0, 16) (-20.3, 0, 16) on bodies 1
fillet "Fillet6" radius 1 2 edges at (-20.3, 28.5, 36.3) (40.9, 28.5, 36.3) on bodies 2
fillet "Fillet7" radius 1 5 edges at (40.9, 56, 36.3) (10.3, 57, 36.3) (40.9, 57, 16) (-20.3, 56, 36.3) (-20.3, 57, 16) on bodies 3
sketch "Sketch17" plane through (0, 57, 0) normal (0, 1, 0) x (-1, 0, 0)
  circle A0 centre (13.365, 30.08) radius 2.7
  circle A1 centre (-29.645, 2.08) radius 2.7
  line L0 (19.3, -4.3) -> (19.3, 35.3)
  line L1 (19.3, 35.3) -> (-39.9, 35.3)
  line L2 (-39.9, 35.3) -> (-39.9, -4.3)
  line L3 (-39.9, -4.3) -> (19.3, -4.3)
  circle A2 centre (-29.635, 30.08) radius 2.7
  circle A3 centre (13.34, 2.07) radius 2.7
  arc A4 (-7.2395, -2.26) -> (-7.2395, 4.3) centre (-7.3209, 1.02) ccw
  line L4 (-13.1801, 4.3) -> (-7.2395, 4.3)
  arc A5 (-13.1801, 4.3) -> (-13.1801, -2.26) centre (-13.0999, 1.02) ccw
  line L5 (-7.2395, -2.26) -> (-13.1801, -2.26)
  line L6 (-25, 20) -> (5, 20) construction
  line L7 (5, 20) -> (5, 25) construction
  line L8 (5, 25) -> (-25, 25) construction
  line L9 (-25, 25) -> (-25, 20) construction
  dimension "d128" = 2.8
extrude "Extrude17" cut sketch "Sketch17" against normal blind 2 contours A4 L4 A5 L5 bodies 3
sketch "Sketch18" plane through (0, 57, 0) normal (0, 1, 0) x (-1, 0, 0)
  line L0 (-7.2395, -2.26) -> (-13.1801, -2.26)
  arc A0 (-13.1801, 4.3) -> (-13.1801, -2.26) centre (-13.0999, 1.02) ccw
  line L1 (-13.1801, 4.3) -> (-7.2395, 4.3)
  arc A1 (-7.2395, -2.26) -> (-7.2395, 4.3) centre (-7.3209, 1.02) ccw
  circle A2 centre (13.365, 30.08) radius 2.7
  circle A3 centre (-29.645, 2.08) radius 2.7
  line L2 (19.3, -4.3) -> (19.3, 35.3)
  line L3 (19.3, 35.3) -> (-39.9, 35.3)
  line L4 (-39.9, 35.3) -> (-39.9, -4.3)
  line L5 (-39.9, -4.3) -> (19.3, -4.3)
  circle A4 centre (-29.635, 30.08) radius 2.7
  circle A5 centre (13.34, 2.07) radius 2.7
sketch "Sketch19" plane through (0, 57, 0) normal (0, 1, 0) x (-1, 0, 0)
sketch "Sketch20" plane through (0, 0, -4.3) normal (0, 0, -1) x (1, 0, 0)
  line L0 (-20.3, -2) -> (-20.3, -55)
  line L1 (-20.3, -55) -> (40.9, -55)
  line L2 (40.9, -55) -> (40.9, -2)
  line L3 (40.9, -2) -> (-20.3, -2)
equation "d39 = '103450 3.7v 2000mah'"
equation "d114 = 'ESP-32 C6 is not in the enclosure as its going to be free floating inside for ease of debugging and assembly'"
equation "d129 = 'AirLog-E'"
named bodies: "Front Plate", "Main Enclosure", "Back Plate"
